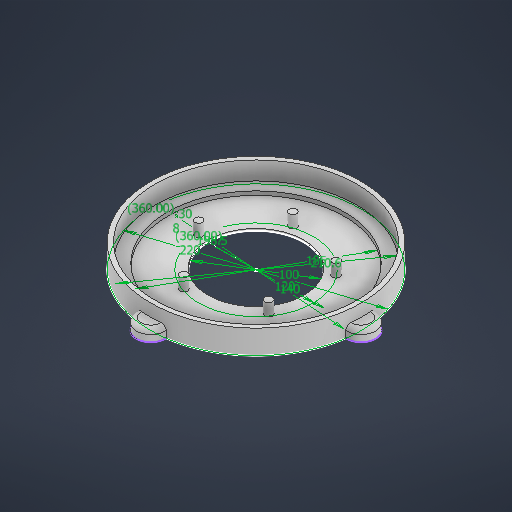
# Autodesk Inventor part: GroundPlate_Aperatus
Saved by Autodesk Inventor 2026.2 (Build 302298000, 298)
## iProperties
Created: 2025-12-30
Part Number: GroundPlate_Aperatus
Material: Generic
Document SubType Name: Modeling
Designer: Cobble
Density: 1 g/cm^3
Appearance: Default
Author: Cobble
Autodesk Inventor part; units mm, degrees
ref_plane "YZ Plane" through (0, 0, 0) normal (1, 0, 0) x (0, 1, 0)
ref_plane "XZ Plane" through (0, 0, 0) normal (0, 1, 0) x (-1, 0, 0)
ref_plane "XY Plane" through (0, 0, 0) normal (0, 0, 1) x (1, 0, 0)
sketch "Sketch1" plane through (0, 0, 0) normal (0, 0, 1) x (1, 0, 0)
  circle A0 centre (0, 0) radius 50
  circle A1 centre (0, 0) radius 60
  circle A2 centre (0, 0) radius 70
  circle A3 centre (-60, 0) radius 4
  circle A4 centre (-18.541, -57.0634) radius 4
  circle A5 centre (48.541, -35.2671) radius 4
  circle A6 centre (48.541, 35.2671) radius 4
  circle A7 centre (-18.541, 57.0634) radius 4
  circle A8 centre (0, 0) radius 105.3
  circle A9 centre (0, 0) radius 92.5
  circle A10 centre (0, 0) radius 99.25 construction
  line L0 (0, 0) -> (-99.25, 0) construction
  circle A11 centre (0, 0) radius 110
  circle A12 centre (-110, 0) radius 15
  circle A13 centre (0, -110) radius 15
  circle A14 centre (110, 0) radius 15
  circle A15 centre (0, 110) radius 15
  point P0 (-14.9651, -108.9773)
  point P1 (14.9651, -108.9773)
  point P2 (108.9773, -14.9651)
  point P3 (108.9773, 14.9651)
  point P4 (-14.9651, 108.9773)
  point P5 (14.9651, 108.9773)
  point P6 (-108.9773, -14.9651)
  point P7 (-108.9773, 14.9651)
  dimension "d1" = 120
  dimension "d14" = 198.5
  dimension "d22" = 220
  dimension "d0" = 100
  dimension "d2" = 140
  dimension "d3" = 8
  dimension "d6" = 360
  dimension "d12" = 210.6
  dimension "d13" = 185
  dimension "d25" = 30
  dimension "d28" = 360
  constraints: 13 centre point, 7 coincident, 2 end point, 2 horizontal alignment, 1 horizontal, 27 other
  measures "d0" diameter of A0
  measures "d2" diameter of A2
  measures "d3" diameter of A3
  measures "d12" diameter of A8
  measures "d13" diameter of A9
  measures "d25" diameter of A12
extrude "Extrusion1" add sketch "Sketch1" along normal blind 2 contours A1 A5 A4 A3 A7 A6 | A2 | A9
extrude "Extrusion2" add sketch "Sketch1" along normal blind 15 contours A6 A1 | A1 A6 | A5 A1 | A1 A5 | A7 A1 | A1 A7 | A4 A1 | A1 A4 | A3 A1 | A1 A3
extrude "Extrusion3" add sketch "Sketch1" along normal blind 6 contours A8 A14 | A14 A8 A13 A12 A15 | A15 A8 | A8 A13 | A12 A8
extrude "Extrusion4" add sketch "Sketch1" along normal blind 12 contours A8 A14 A11 | A8 A15 A11 A14 | A14 A11 A13 A8 | A8 A15 A11 | A14 A11 | A13 A11 A8 | A8 A12 A11 A15 | A11 A15 | A13 A11 A12 A8 | A13 A11 | A8 A12 A11 | A11 A12
fillet "Fillet1" radius 5 4 edges at (-125, 0, 12) (0, -125, 12) (125, 0, 12) (0, 125, 12)
extrude "Extrusion5" add sketch "Sketch1" along normal blind 25 contours A8 A14 A11 | A8 A15 A11 A14 | A14 A11 A13 A8 | A8 A15 A11 | A13 A11 A8 | A8 A12 A11 A15 | A13 A11 A12 A8 | A8 A12 A11
body "Solid1"
